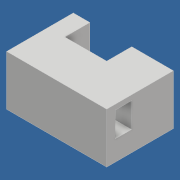
# Autodesk Inventor part: Part2
Saved by Autodesk Inventor 2018 (Build 220112000, 112)
## iProperties
Created: 2017-12-05
Part Number: Part2
Material: Generic
Document SubType Name: Modeling
Designer: 232963
Density: 1 g/cm^3
Appearance: Default
Author: 232963
Autodesk Inventor part; units mm, degrees
ref_plane "YZ Plane" through (0, 0, 0) normal (1, 0, 0) x (0, 1, 0)
ref_plane "XZ Plane" through (0, 0, 0) normal (0, 1, 0) x (-1, 0, 0)
ref_plane "XY Plane" through (0, 0, 0) normal (0, 0, 1) x (1, 0, 0)
sketch "Sketch1" plane through (0, 0, 0) normal (0, 0, 1) x (1, 0, 0)
  line L0 (35.6681, 35) -> (35.6681, -5)
  line L1 (35.6681, -5) -> (-24.3319, -5)
  line L2 (-24.3319, -5) -> (-24.3319, 35)
  line L3 (10.6681, 35) -> (10.6681, 20)
  line L4 (10.6681, 20) -> (-14.3319, 20)
  line L5 (-14.3319, 20) -> (-14.3319, 35)
  line L6 (-24.3319, 35) -> (-14.3319, 35)
  line L7 (10.6681, 35) -> (35.6681, 35)
  point P0 (0, 0)
  dimension "d0" = 60
  dimension "d1" = 40
  dimension "d2" = 10
  dimension "d3" = 15
  dimension "d4" = 25
  constraints: 16 end point, 4 parallel, 2 horizontal, 2 perpendicular
  measures "d0" distance of L0.end L1.end
  measures "d1" distance of L0.start L0.end
  measures "d2" distance of L2.end L5.end
  measures "d3" distance of L4.end L5.end
  measures "d4" distance of L3.start L0.start
extrude "Extrusion1" add sketch "Sketch1" along normal blind 30
sketch "Sketch2" plane through (35.6681, -5, 0) normal (1, 0, 0) x (0, 0, -1)
  line L0 (-27, 15) -> (-12, 15)
  line L1 (-12, 15) -> (-12, 5)
  line L2 (-12, 5) -> (-27, 5)
  line L3 (-27, 5) -> (-27, 15)
  line L4 (0, 0) -> (-30, 0) projected
  line L5 (-30, 0) -> (-30, 40) projected
  point P0 (0, 5)
  dimension "d7" = 15
  dimension "d8" = 10
  dimension "d9" = 5
  dimension "d10" = 3
  constraints: 8 end point, 2 parallel, 1 horizontal, 1 perpendicular
  measures "d7" distance of L0.start L0.end
  measures "d8" distance of L2.end L0.start
  measures "d9" distance between parallel lines of L4 L2
  measures "d10" distance between parallel lines of L5 L3
extrude "Extrusion2" cut sketch "Sketch2" against normal blind 60
body "Solid1"
